Autodesk Fusion 360 part; units mm, degrees
(part 8 of 11)
  line L1134 (-0.172, -45.5718) -> (-0.1441, -45.6166)
  line L1135 (0.0223, -214.4938) -> (0.0013, -214.5276)
  line L1136 (14.483, -219.9371) -> (14.5191, -219.9534)
  line L1137 (-0.1969, -194.4741) -> (-0.2187, -194.5222)
  line L1138 (6.02, -212.839) -> (3.3593, -215.4997)
  line L1139 (0.0013, -194.5276) -> (-0.0174, -194.5626)
  line L1140 (14.4479, -219.9183) -> (14.483, -219.9371)
  line L1141 (-0.0683, -45.2866) -> (-0.0593, -45.3253)
  line L1142 (-0.0478, -45.3633) -> (-0.0338, -45.4005)
  line L1143 (19.8859, -185.7366) -> (19.9198, -185.7004)
  line L1144 (-0.2646, -214.6736) -> (-0.2732, -214.7258)
  line L1145 (14.7482, -220.1997) -> (18.42, -220.1997)
  line L1146 (9.713, -186.0997) -> (7.0807, -186.0997)
  line L1147 (-0.2786, -45.2189) -> (-0.2732, -45.2736)
  line L1148 (-0.0683, -214.7127) -> (-0.0748, -214.7519)
  line L1149 (19.9083, -185.2866) -> (19.9148, -185.2474)
  line L1150 (14.7514, -219.9997) -> (18.42, -219.9997)
  line L1151 (-0.0338, -214.5988) -> (-0.0478, -214.636)
  line L1152 (-0.0787, -45.2079) -> (-0.0748, -45.2474)
  line L1153 (14.4142, -219.8974) -> (14.4479, -219.9183)
  line L1154 (0.0454, -194.4616) -> (0.0223, -194.4938)
  line L1155 (-0.0748, -45.2474) -> (-0.0683, -45.2866)
  line L1156 (-0.1133, -45.6596) -> (-0.0798, -45.7004)
  line L1157 (14.3819, -219.8742) -> (14.4142, -219.8974)
  line L1158 (19.92, -218.4997) -> (19.92, -214.8311)
  line L1159 (-0.08, -45.0997) -> (-0.0787, -45.2079)
  line L1160 (0.0706, -45.5685) -> (0.0978, -45.5975)
  line L1161 (-0.28, -45.1009) -> (-0.2786, -45.2189)
  line L1162 (0.0454, -45.5378) -> (0.0706, -45.5685)
  line L1163 (-0.0593, -194.674) -> (-0.0683, -194.7127)
  line L1164 (-0.0798, -45.7004) -> (-0.0459, -45.7366)
  line L1165 (-0.2373, -194.5717) -> (-0.2526, -194.6222)
  line L1166 (-0.0798, -194.2989) -> (-0.1133, -194.3397)
  line L1167 (0.0978, -194.4019) -> (0.0706, -194.4308)
  line L1168 (14.3222, -219.8219) -> (14.3512, -219.849)
  line L1169 (0.0013, -45.4717) -> (0.0223, -45.5055)
  line L1170 (-0.0478, -194.636) -> (-0.0593, -194.674)
  line L1171 (-0.0683, -194.7127) -> (-0.0748, -194.7519)
  line L1172 (19.8574, -185.4367) -> (19.8738, -185.4005)
  line L1173 (9.713, -186.0997) -> (7.0807, -186.0997)
  line L1174 (14.594, -220.1843) -> (14.6461, -220.1929)
  line L1175 (14.7117, -219.9984) -> (14.7514, -219.9997)
  line L1176 (16.5635, -215.2997) -> (14.02, -212.7562)
  line L1177 (20.1186, -185.2189) -> (20.12, -185.1009)
  line L1178 (19.92, -218.4997) -> (19.92, -214.8311)
  line L1179 (19.8993, -185.3253) -> (19.9083, -185.2866)
  line L1180 (0.0223, -194.4938) -> (0.0013, -194.5276)
  line L1181 (-0.0478, -194.636) -> (-0.0593, -194.674)
  line L1182 (-0.2646, -194.6736) -> (-0.2732, -194.7258)
  line L1183 (-0.0338, -194.5988) -> (-0.0478, -194.636)
  line L1184 (9.7959, -185.8997) -> (7.1635, -185.8997)
  line L1185 (-0.0748, -194.7519) -> (-0.0787, -194.7914)
  line L1186 (20.12, -218.4997) -> (20.12, -214.8278)
  line L1187 (-0.1133, -194.3397) -> (-0.1441, -194.3827)
  line L1188 (6.02, -192.839) -> (3.3593, -195.4997)
  line L1189 (19.7946, -185.5378) -> (19.8177, -185.5055)
  line L1190 (3.6807, -182.6997) -> (1.72, -182.6997)
  circle A77 centre (9.92, -209.9997) radius 2.1
  arc A78 (13.1828, -217.9997) -> (12.9, -218.6825) centre (13.1828, -218.3997) ccw
  line L1191 (19.9198, -185.7004) -> (19.9533, -185.6596)
  line L1192 (1.72, -177.2997) -> (3.6807, -177.2997)
  line L1193 (19.8738, -185.4005) -> (19.8878, -185.3633)
  line L1194 (13.82, -210.1995) -> (13.6201, -209.9997)
  line L1195 (1.92, -182.4997) -> (1.92, -177.4997)
  line L1196 (1.72, -182.6997) -> (1.72, -177.2997)
  line L1197 (13.6201, -209.9997) -> (13.82, -209.7998)
  line L1198 (-0.1133, -214.3397) -> (-0.1441, -214.3827)
  line L1199 (-0.1441, -214.3827) -> (-0.172, -214.4275)
  line L1200 (-0.0683, -214.7127) -> (-0.0748, -214.7519)
  line L1201 (-0.0683, -194.7127) -> (-0.0748, -194.7519)
  line L1202 (20.0926, -185.3771) -> (20.1046, -185.3257)
  line L1203 (16.4807, -215.4997) -> (13.82, -212.839)
  line L1204 (-0.0459, -214.2627) -> (-0.0798, -214.2989)
  line L1205 (1.72, -182.6997) -> (1.72, -177.2997)
  line L1206 (19.9148, -185.2474) -> (19.9187, -185.2079)
  line L1207 (20.0587, -185.4771) -> (20.0773, -185.4277)
  line L1208 (14.02, -212.7562) -> (14.02, -210.1167)
  line L1209 (19.9148, -185.2474) -> (19.9187, -185.2079)
  line L1210 (-0.0787, -214.7914) -> (-0.08, -214.8997)
  line L1211 (19.8878, -185.3633) -> (19.8993, -185.3253)
  line L1212 (9.7981, -214.0997) -> (9.9208, -213.977)
  line L1213 (-0.2187, -194.5222) -> (-0.2373, -194.5717)
  line L1214 (-0.2786, -214.7804) -> (-0.28, -214.8985)
  line L1215 (0.0223, -194.4938) -> (0.0013, -194.5276)
  line L1216 (1.92, -177.4997) -> (3.7635, -177.4997)
  line L1217 (0.0978, -194.4019) -> (0.0706, -194.4308)
  line L1218 (3.7635, -182.4997) -> (1.92, -182.4997)
  line L1219 (-0.0787, -194.7914) -> (-0.08, -194.8997)
  line L1220 (-0.0787, -194.7914) -> (-0.08, -194.8997)
  line L1221 (-0.2373, -214.5717) -> (-0.2526, -214.6222)
  line L1222 (19.9533, -185.6596) -> (19.9841, -185.6166)
  line L1223 (10.127, -213.8997) -> (12.7593, -213.8997)
  line L1224 (0.0013, -194.5276) -> (-0.0174, -194.5626)
  line L1225 (-0.1969, -214.4741) -> (-0.2187, -214.5222)
  line L1226 (0.0706, -194.4308) -> (0.0454, -194.4616)
  line L1227 (14.02, -210.1167) -> (13.903, -209.9997)
  line L1228 (19.9083, -185.2866) -> (19.9148, -185.2474)
  line L1229 (-0.0338, -194.5988) -> (-0.0478, -194.636)
  line L1230 (20.1046, -185.3257) -> (20.1132, -185.2736)
  line L1231 (3.6807, -162.6997) -> (1.72, -162.6997)
  line L1232 (-0.0174, -194.5626) -> (-0.0338, -194.5988)
  line L1233 (-0.0478, -214.636) -> (-0.0593, -214.674)
  line L1234 (-0.172, -214.4275) -> (-0.1969, -214.4741)
  line L1235 (-0.0748, -194.7519) -> (-0.0787, -194.7914)
  line L1236 (0.0706, -214.4308) -> (0.0454, -214.4616)
  line L1237 (-0.0174, -214.5626) -> (-0.0338, -214.5988)
  line L1238 (9.7152, -213.8997) -> (9.92, -213.6949)
  line L1239 (-0.2732, -194.7258) -> (-0.2786, -194.7804)
  line L1240 (19.7694, -185.5685) -> (19.7946, -185.5378)
  circle A79 centre (9.92, -209.9997) radius 2.1
  line L1241 (0.0454, -194.4616) -> (0.0223, -194.4938)
  line L1242 (0.0706, -194.4308) -> (0.0454, -194.4616)
  line L1243 (19.8177, -185.5055) -> (19.8387, -185.4717)
  line L1244 (-0.0593, -214.674) -> (-0.0683, -214.7127)
  line L1245 (3.6807, -182.6997) -> (1.72, -182.6997)
  line L1246 (19.8387, -185.4717) -> (19.8574, -185.4367)
  line L1247 (13.903, -209.9997) -> (14.02, -209.8826)
  line L1248 (-0.0787, -214.7914) -> (-0.08, -214.8997)
  line L1249 (19.9187, -185.2079) -> (19.92, -185.0997)
  line L1250 (9.9208, -213.977) -> (10.0448, -214.0997)
  line L1251 (1.72, -177.2997) -> (3.6807, -177.2997)
  line L1252 (0.0978, -214.4019) -> (0.0706, -214.4308)
  line L1253 (10.127, -213.8997) -> (12.7593, -213.8997)
  line L1254 (1.2372, -192.9797) -> (-0.0459, -194.2627)
  arc A80 (13.1828, -218.1997) -> (13.0414, -218.5411) centre (13.1828, -218.3997) ccw
  line L1255 (1.72, -164.4997) -> (3.3593, -164.4997)
  line L1256 (-0.0593, -214.674) -> (-0.0683, -214.7127)
  line L1257 (3.7635, -202.4997) -> (1.92, -202.4997)
  line L1258 (1.92, -202.4997) -> (1.92, -197.4997)
  line L1259 (20.1132, -185.2736) -> (20.1186, -185.2189)
  line L1260 (14.1831, -219.9656) -> (14.2193, -219.9995)
  line L1261 (0.0013, -214.5276) -> (-0.0174, -214.5626)
  line L1262 (9.7152, -213.8997) -> (9.92, -213.6949)
  line L1263 (0.0454, -214.4616) -> (0.0223, -214.4938)
  line L1264 (-0.0798, -214.2989) -> (-0.1133, -214.3397)
  line L1265 (19.8738, -185.4005) -> (19.8878, -185.3633)
  line L1266 (-0.1441, -194.3827) -> (-0.172, -194.4275)
  line L1267 (20.0773, -185.4277) -> (20.0926, -185.3771)
  line L1268 (19.7694, -185.5685) -> (19.7946, -185.5378)
  line L1269 (1.72, -166.7368) -> (1.72, -164.4997)
  line L1270 (-0.0459, -194.2627) -> (-0.0798, -194.2989)
  line L1271 (-0.2526, -194.6222) -> (-0.2646, -194.6736)
  line L1272 (1.92, -166.7368) -> (1.92, -164.6997)
  arc A81 (1.3786, -166.8782) -> (1.72, -166.7368) centre (1.52, -166.7368) ccw
  line L1273 (13.82, -210.1995) -> (13.6201, -209.9997)
  line L1274 (-0.0478, -214.636) -> (-0.0593, -214.674)
  line L1275 (19.8993, -185.3253) -> (19.9083, -185.2866)
  line L1276 (20.012, -185.5718) -> (20.0369, -185.5252)
  line L1277 (19.8878, -185.3633) -> (19.8993, -185.3253)
  line L1278 (10.0448, -214.0997) -> (12.6765, -214.0997)
  line L1279 (19.8387, -185.4717) -> (19.8574, -185.4367)
  arc A82 (13.1828, -218.1997) -> (13.0414, -218.5411) centre (13.1828, -218.3997) ccw
  line L1280 (12.9, -218.6825) -> (14.1831, -219.9656)
  line L1281 (-0.0748, -214.7519) -> (-0.0787, -214.7914)
  line L1282 (13.6201, -209.9997) -> (13.82, -209.7998)
  line L1283 (19.9841, -185.6166) -> (20.012, -185.5718)
  line L1284 (3.6807, -202.6997) -> (1.72, -202.6997)
  line L1285 (0.0013, -214.5276) -> (-0.0174, -214.5626)
  line L1286 (3.2765, -164.6997) -> (5.82, -167.2432)
  line L1287 (19.9187, -185.2079) -> (19.92, -185.0997)
  line L1288 (3.6807, -162.6997) -> (1.72, -162.6997)
  line L1289 (1.92, -197.4997) -> (3.7635, -197.4997)
  line L1290 (19.8177, -185.5055) -> (19.8387, -185.4717)
  line L1291 (13.82, -212.839) -> (13.82, -210.1995)
  line L1292 (0.0978, -214.4019) -> (0.0706, -214.4308)
  line L1293 (-0.0748, -214.7519) -> (-0.0787, -214.7914)
  line L1294 (20.0369, -185.5252) -> (20.0587, -185.4771)
  arc A83 (1.3786, -166.8782) -> (1.72, -166.7368) centre (1.52, -166.7368) ccw
  line L1295 (19.8574, -185.4367) -> (19.8738, -185.4005)
  line L1296 (1.72, -197.2997) -> (3.6807, -197.2997)
  line L1297 (9.92, -213.6949) -> (10.127, -213.8997)
  line L1298 (-0.2732, -214.7258) -> (-0.2786, -214.7804)
  line L1299 (-0.2786, -194.7804) -> (-0.28, -194.8985)
  line L1300 (1.72, -202.6997) -> (1.72, -197.2997)
  line L1301 (9.92, -213.6949) -> (10.127, -213.8997)
  line L1302 (-0.2187, -214.5222) -> (-0.2373, -214.5717)
  line L1303 (-0.0338, -214.5988) -> (-0.0478, -214.636)
  line L1304 (13.82, -212.839) -> (13.82, -210.1995)
  line L1305 (0.0454, -214.4616) -> (0.0223, -214.4938)
  line L1306 (0.0706, -214.4308) -> (0.0454, -214.4616)
  line L1307 (19.7946, -185.5378) -> (19.8177, -185.5055)
  line L1308 (13.0414, -218.5411) -> (14.3222, -219.8219)
  line L1309 (-0.2526, -214.6222) -> (-0.2646, -214.6736)
  line L1310 (13.0414, -218.5411) -> (14.3222, -219.8219)
  line L1311 (1.72, -206.7368) -> (1.72, -204.4997)
  line L1312 (7.0807, -173.8997) -> (9.713, -173.8997)
  line L1313 (9.713, -166.0997) -> (7.0807, -166.0997)
  arc A84 (1.3786, -206.8782) -> (1.72, -206.7368) centre (1.52, -206.7368) ccw
  line L1314 (-0.2526, -185.3771) -> (-0.2373, -185.4277)
  line L1315 (18.12, -184.4997) -> (18.12, -186.7368)
  line L1316 (19.7422, -185.5975) -> (19.7694, -185.5685)
  line L1317 (16.4807, -215.4997) -> (13.82, -212.839)
  line L1318 (-0.0478, -185.3633) -> (-0.0338, -185.4005)
  arc A85 (17.92, -186.7368) -> (18.6028, -187.0197) centre (18.32, -186.7368) ccw
  line L1319 (15.42, -218.1997) -> (13.1828, -218.1997)
  line L1320 (1.72, -184.4997) -> (3.3593, -184.4997)
  line L1321 (1.3786, -213.1211) -> (0.0978, -214.4019)
  arc A86 (1.3786, -206.8782) -> (1.72, -206.7368) centre (1.52, -206.7368) ccw
  line L1322 (9.7959, -165.8997) -> (7.1635, -165.8997)
  line L1323 (-0.28, -185.1009) -> (-0.2786, -185.2189)
  line L1324 (1.2372, -212.9797) -> (-0.0459, -214.2627)
  line L1325 (-0.0174, -214.5626) -> (-0.0338, -214.5988)
  line L1326 (18.12, -184.4997) -> (18.12, -186.7368)
  line L1327 (6.02, -210.1995) -> (6.02, -212.839)
  line L1328 (17.92, -184.6997) -> (17.92, -186.7368)
  line L1329 (0.0223, -214.4938) -> (0.0013, -214.5276)
  line L1330 (-0.2187, -185.4771) -> (-0.1969, -185.5252)
  arc A87 (18.12, -186.7368) -> (18.4614, -186.8782) centre (18.32, -186.7368) ccw
  line L1331 (1.92, -184.6997) -> (3.2765, -184.6997)
  line L1332 (12.7593, -213.8997) -> (15.42, -216.5603)
  line L1333 (12.7593, -213.8997) -> (15.42, -216.5603)
  arc A88 (1.2372, -207.0197) -> (1.92, -206.7368) centre (1.52, -206.7368) ccw
  line L1334 (-0.172, -185.5718) -> (-0.1441, -185.6166)
  line L1335 (18.4614, -186.8782) -> (19.7422, -185.5975)
  line L1336 (3.2765, -204.6997) -> (5.82, -207.2432)
  line L1337 (1.72, -164.4997) -> (3.3593, -164.4997)
  line L1338 (1.3786, -213.1211) -> (0.0978, -214.4019)
  line L1339 (1.72, -166.7368) -> (1.72, -164.4997)
  line L1340 (12.6765, -214.0997) -> (15.22, -216.6432)
  line L1341 (1.92, -204.6997) -> (3.2765, -204.6997)
  line L1342 (1.72, -197.2997) -> (3.6807, -197.2997)
  line L1343 (18.4614, -186.8782) -> (19.7422, -185.5975)
  line L1344 (-0.2732, -185.2736) -> (-0.2646, -185.3257)
  line L1345 (5.82, -212.7562) -> (3.2765, -215.2997)
  line L1346 (-0.0338, -185.4005) -> (-0.0174, -185.4367)
  line L1347 (0.0978, -205.5975) -> (1.3786, -206.8782)
  line L1348 (1.72, -202.6997) -> (1.72, -197.2997)
  line L1349 (0.0223, -185.5055) -> (0.0454, -185.5378)
  line L1350 (4.42, -216.5603) -> (7.0807, -213.8997)
  line L1351 (3.3593, -164.4997) -> (6.02, -167.1603)
  line L1352 (-0.0748, -185.2474) -> (-0.0683, -185.2866)
  line L1353 (7.0807, -186.0997) -> (3.6807, -182.6997)
  line L1354 (15.22, -217.9997) -> (13.1828, -217.9997)
  line L1355 (3.3593, -164.4997) -> (6.02, -167.1603)
  line L1356 (6.02, -210.1995) -> (6.02, -212.839)
  line L1357 (7.0807, -166.0997) -> (3.6807, -162.6997)
  line L1358 (1.92, -164.6997) -> (3.2765, -164.6997)
  line L1359 (3.6807, -202.6997) -> (1.72, -202.6997)
  line L1360 (7.0807, -166.0997) -> (3.6807, -162.6997)
  line L1361 (15.42, -218.1997) -> (13.1828, -218.1997)
  line L1362 (7.1635, -165.8997) -> (3.7635, -162.4997)
  arc A89 (18.12, -186.7368) -> (18.4614, -186.8782) centre (18.32, -186.7368) ccw
  line L1363 (19.7422, -185.5975) -> (19.7694, -185.5685)
  line L1364 (18.6028, -187.0197) -> (19.8859, -185.7366)
  line L1365 (-0.2373, -185.4277) -> (-0.2187, -185.4771)
  line L1366 (3.7635, -197.4997) -> (7.1635, -194.0997)
  line L1367 (-0.2646, -185.3257) -> (-0.2526, -185.3771)
  line L1368 (1.72, -186.7368) -> (1.72, -184.4997)
  arc A90 (6.94, -218.6825) -> (6.6572, -217.9997) centre (6.6572, -218.3997) ccw
  line L1369 (7.0807, -186.0997) -> (3.6807, -182.6997)
  line L1370 (0.0013, -185.4717) -> (0.0223, -185.5055)
  line L1371 (5.5178, -219.8219) -> (6.7986, -218.5411)
  line L1372 (9.92, -186.3066) -> (9.713, -186.0997)
  line L1373 (-0.28, -214.8985) -> (-0.28, -218.4997)
  line L1374 (16.0765, -182.4997) -> (12.6765, -185.8997)
  arc A91 (6.7986, -218.5411) -> (6.6572, -218.1997) centre (6.6572, -218.3997) ccw
  line L1375 (1.72, -204.4997) -> (3.3593, -204.4997)
  line L1376 (4.62, -216.6432) -> (7.1635, -214.0997)
  line L1377 (0.0978, -205.5975) -> (1.3786, -206.8782)
  line L1378 (5.5178, -219.8219) -> (6.7986, -218.5411)
  line L1379 (3.6807, -197.2997) -> (7.0807, -193.8997)
  line L1380 (1.72, -206.7368) -> (1.72, -204.4997)
  line L1381 (-0.0683, -185.2866) -> (-0.0593, -185.3253)
  line L1382 (1.92, -206.7368) -> (1.92, -204.6997)
  line L1383 (13.82, -189.7998) -> (13.82, -187.1603)
  line L1384 (6.6572, -217.9997) -> (4.62, -217.9997)
  line L1385 (0.0978, -185.5975) -> (1.3786, -186.8782)
  line L1386 (7.1635, -185.8997) -> (3.7635, -182.4997)
  line L1387 (6.6572, -218.1997) -> (4.42, -218.1997)
  arc A92 (6.7986, -218.5411) -> (6.6572, -218.1997) centre (6.6572, -218.3997) ccw
  line L1388 (-0.0478, -165.3633) -> (-0.0338, -165.4005)
  line L1389 (4.62, -217.9997) -> (4.62, -216.6432)
  line L1390 (4.42, -218.1997) -> (4.42, -216.5603)
  line L1391 (-0.08, -214.8997) -> (-0.08, -218.4997)
  line L1392 (-0.0593, -165.3253) -> (-0.0478, -165.3633)
  line L1393 (-0.0787, -185.2079) -> (-0.0748, -185.2474)
  line L1394 (1.72, -204.4997) -> (3.3593, -204.4997)
  line L1395 (-0.2786, -185.2189) -> (-0.2732, -185.2736)
  line L1396 (-0.0174, -185.4367) -> (0.0013, -185.4717)
  line L1397 (-0.0478, -185.3633) -> (-0.0338, -185.4005)
  line L1398 (9.92, -186.0238) -> (9.7959, -185.8997)
  line L1399 (0.0013, -185.4717) -> (0.0223, -185.5055)
  line L1400 (7.0807, -206.0997) -> (3.6807, -202.6997)
  line L1401 (-0.0338, -165.4005) -> (-0.0174, -165.4367)
  line L1402 (10.0441, -185.8997) -> (9.92, -186.0238)
  line L1403 (-0.1133, -185.6596) -> (-0.0798, -185.7004)
  line L1404 (16.1593, -182.6997) -> (12.7593, -186.0997)
  line L1405 (-0.1441, -165.6166) -> (-0.1133, -165.6596)
  line L1406 (7.1635, -205.8997) -> (3.7635, -202.4997)
  line L1407 (12.6765, -185.8997) -> (10.0441, -185.8997)
  line L1408 (0.0223, -185.5055) -> (0.0454, -185.5378)
  line L1409 (1.72, -184.4997) -> (3.3593, -184.4997)
  line L1410 (-0.0683, -165.2866) -> (-0.0593, -165.3253)
  line L1411 (6.6572, -218.1997) -> (4.42, -218.1997)
  line L1412 (13.82, -190.1995) -> (13.6201, -189.9997)
  line L1413 (-0.1969, -185.5252) -> (-0.172, -185.5718)
  line L1414 (0.0706, -165.5685) -> (0.0978, -165.5975)
  line L1415 (1.92, -186.7368) -> (1.92, -184.6997)
  line L1416 (10.127, -186.0997) -> (9.92, -186.3066)
  line L1417 (-0.0683, -165.2866) -> (-0.0593, -165.3253)
  line L1418 (-0.08, -165.0997) -> (-0.0787, -165.2079)
  line L1419 (-0.1441, -185.6166) -> (-0.1133, -185.6596)
  line L1420 (0.0454, -185.5378) -> (0.0706, -185.5685)
  line L1421 (4.42, -218.1997) -> (4.42, -216.5603)
  line L1422 (13.82, -190.1995) -> (13.6201, -189.9997)
  line L1423 (-0.28, -165.1009) -> (-0.2786, -165.2189)
  line L1424 (-0.0787, -185.2079) -> (-0.0748, -185.2474)
  line L1425 (3.3593, -184.4997) -> (6.02, -187.1603)
  line L1426 (13.903, -189.9997) -> (14.02, -189.8826)
  line L1427 (-0.0787, -165.2079) -> (-0.0748, -165.2474)
  line L1428 (-0.0174, -185.4367) -> (0.0013, -185.4717)
  line L1429 (0.0978, -185.5975) -> (1.3786, -186.8782)
  line L1430 (5.6207, -219.9995) -> (5.6569, -219.9656)
  line L1431 (-0.0593, -185.3253) -> (-0.0478, -185.3633)
  line L1432 (5.2837, -219.9674) -> (5.3209, -219.9534)
  line L1433 (7.1635, -174.0997) -> (9.7959, -174.0997)
  line L1434 (-0.0478, -205.3633) -> (-0.0338, -205.4005)
  line L1435 (-0.2732, -205.2736) -> (-0.2646, -205.3257)
  line L1436 (14.02, -190.1167) -> (13.903, -189.9997)
  line L1437 (13.6201, -189.9997) -> (13.82, -189.7998)
  line L1438 (12.7593, -186.0997) -> (10.127, -186.0997)
  line L1439 (16.1593, -182.6997) -> (12.7593, -186.0997)
  line L1440 (-0.2373, -205.4277) -> (-0.2187, -205.4771)
  line L1441 (0.0454, -165.5378) -> (0.0706, -165.5685)
  line L1442 (-0.172, -165.5718) -> (-0.1441, -165.6166)
  line L1443 (-0.0174, -165.4367) -> (0.0013, -165.4717)
  line L1444 (4.42, -216.5603) -> (7.0807, -213.8997)
  line L1445 (13.82, -187.1603) -> (16.4807, -184.4997)
  line L1446 (3.2765, -184.6997) -> (5.82, -187.2432)
  line L1447 (0.0223, -165.5055) -> (0.0454, -165.5378)
  line L1448 (12.7593, -186.0997) -> (10.127, -186.0997)
  line L1449 (-0.2786, -205.2189) -> (-0.2732, -205.2736)
  line L1450 (-0.0593, -185.3253) -> (-0.0478, -185.3633)
  line L1451 (5.4455, -220.1165) -> (5.4921, -220.0916)
  line L1452 (-0.08, -214.8997) -> (-0.08, -218.4997)
  line L1453 (-0.0683, -205.2866) -> (-0.0593, -205.3253)
  line L1454 (-0.0787, -165.2079) -> (-0.0748, -165.2474)
  line L1455 (-0.1133, -165.6596) -> (-0.0798, -165.7004)
  line L1456 (-0.0748, -205.2474) -> (-0.0683, -205.2866)
  line L1457 (-0.0174, -205.4367) -> (0.0013, -205.4717)
  line L1458 (3.3593, -204.4997) -> (6.02, -207.1603)
  line L1459 (-0.0748, -165.2474) -> (-0.0683, -165.2866)
  line L1460 (-0.0459, -185.7366) -> (1.2372, -187.0197)
  line L1461 (-0.2187, -165.4771) -> (-0.1969, -165.5252)
  line L1462 (-0.08, -185.0997) -> (-0.0787, -185.2079)
  line L1463 (3.3593, -184.4997) -> (6.02, -187.1603)
  circle A93 centre (9.92, -189.9997) radius 2.1
  line L1464 (13.82, -189.7998) -> (13.82, -187.1603)
  line L1465 (-0.0338, -205.4005) -> (-0.0174, -205.4367)
  line L1466 (0.0706, -185.5685) -> (0.0978, -185.5975)
  line L1467 (5.0918, -220.1997) -> (5.1413, -220.198)
  line L1468 (-0.2526, -165.3771) -> (-0.2373, -165.4277)
  line L1469 (6.02, -192.839) -> (3.3593, -195.4997)
  line L1470 (-0.0748, -185.2474) -> (-0.0683, -185.2866)
  line L1471 (0.0223, -165.5055) -> (0.0454, -165.5378)
  line L1472 (-0.0798, -185.7004) -> (-0.0459, -185.7366)
  line L1473 (13.82, -187.1603) -> (16.4807, -184.4997)
  line L1474 (-0.08, -185.0997) -> (-0.0787, -185.2079)
  line L1475 (9.92, -186.3066) -> (9.713, -186.0997)
  line L1476 (-0.0683, -185.2866) -> (-0.0593, -185.3253)
  line L1477 (1.72, -186.7368) -> (1.72, -184.4997)
  line L1478 (-0.0748, -205.2474) -> (-0.0683, -205.2866)
  line L1479 (-0.0338, -185.4005) -> (-0.0174, -185.4367)
  line L1480 (-0.0174, -165.4367) -> (0.0013, -165.4717)
  line L1481 (0.0454, -185.5378) -> (0.0706, -185.5685)
  line L1482 (9.713, -166.0997) -> (7.0807, -166.0997)
  line L1483 (0.0706, -185.5685) -> (0.0978, -185.5975)
  circle A94 centre (9.92, -189.9997) radius 2.1
  line L1484 (14.02, -189.8826) -> (14.02, -187.2432)
  line L1485 (0.0454, -165.5378) -> (0.0706, -165.5685)
  line L1486 (14.02, -187.2432) -> (16.5635, -184.6997)
  line L1487 (-0.172, -205.5718) -> (-0.1441, -205.6166)
  line L1488 (-0.0593, -165.3253) -> (-0.0478, -165.3633)
  line L1489 (-0.2646, -205.3257) -> (-0.2526, -205.3771)
  line L1490 (13.6201, -189.9997) -> (13.82, -189.7998)
  line L1491 (10.127, -186.0997) -> (9.92, -186.3066)
  line L1492 (16.4807, -184.4997) -> (18.12, -184.4997)
  line L1493 (5.207, -219.988) -> (5.2457, -219.979)
  line L1494 (0.0706, -205.5685) -> (0.0978, -205.5975)
  line L1495 (-0.0748, -165.2474) -> (-0.0683, -165.2866)
  line L1496 (16.5635, -184.6997) -> (17.92, -184.6997)
  line L1497 (-0.0338, -165.4005) -> (-0.0174, -165.4367)
  line L1498 (-0.0593, -205.3253) -> (-0.0478, -205.3633)
  line L1499 (16.4807, -184.4997) -> (18.12, -184.4997)
  line L1500 (5.3921, -219.9183) -> (5.4258, -219.8974)
  line L1501 (3.6807, -197.2997) -> (7.0807, -193.8997)
  line L1502 (7.0807, -173.8997) -> (9.713, -173.8997)
  line L1503 (5.1678, -219.9945) -> (5.207, -219.988)
  line L1504 (12.7593, -146.0997) -> (10.127, -146.0997)
  line L1505 (10.0448, -145.8997) -> (9.9208, -146.0223)
  line L1506 (9.92, -146.3044) -> (9.7152, -146.0997)
  line L1507 (0.0223, -105.5055) -> (0.0454, -105.5378)
  line L1508 (-0.0593, -105.3253) -> (-0.0478, -105.3633)
  line L1509 (-0.172, -105.5718) -> (-0.1441, -105.6166)
  line L1510 (-0.0174, -105.4367) -> (0.0013, -105.4717)
  line L1511 (12.6765, -145.8997) -> (10.0448, -145.8997)
  line L1512 (-0.0787, -105.2079) -> (-0.0748, -105.2474)
  line L1513 (0.0454, -105.5378) -> (0.0706, -105.5685)
  line L1514 (9.9208, -146.0223) -> (9.7981, -145.8997)
  arc A95 (13.1828, -137.9997) -> (12.9, -138.6825) centre (13.1828, -138.3997) ccw
  arc A96 (13.0414, -141.4582) -> (13.1828, -141.7997) centre (13.1828, -141.5997) ccw
  line L1515 (0.0454, -105.5378) -> (0.0706, -105.5685)
  line L1516 (-0.2786, -105.2189) -> (-0.2732, -105.2736)
  line L1517 (0.0706, -105.5685) -> (0.0978, -105.5975)
  line L1518 (0.0013, -105.4717) -> (0.0223, -105.5055)
  line L1519 (10.127, -146.0997) -> (9.92, -146.3044)
  line L1520 (-0.0798, -105.7004) -> (-0.0459, -105.7366)
  line L1521 (-0.2187, -105.4771) -> (-0.1969, -105.5252)
  line L1522 (-0.2373, -105.4277) -> (-0.2187, -105.4771)
  line L1523 (14.1831, -140.0337) -> (12.9, -141.3168)
  line L1524 (14.02, -147.2432) -> (16.5635, -144.6997)
  line L1525 (-0.0593, -105.3253) -> (-0.0478, -105.3633)
  line L1526 (12.9, -138.6825) -> (14.1831, -139.9656)
  line L1527 (-0.28, -105.1009) -> (-0.2786, -105.2189)
  arc A97 (13.1828, -138.1997) -> (13.0414, -138.5411) centre (13.1828, -138.3997) ccw
  line L1528 (0.0013, -105.4717) -> (0.0223, -105.5055)
  line L1529 (15.42, -143.439) -> (12.7593, -146.0997)
  line L1530 (-0.0478, -105.3633) -> (-0.0338, -105.4005)
  line L1531 (-0.2646, -105.3257) -> (-0.2526, -105.3771)
  line L1532 (-0.2526, -105.3771) -> (-0.2373, -105.4277)
  line L1533 (9.92, -146.3044) -> (9.7152, -146.0997)
  arc A98 (12.9, -141.3168) -> (13.1828, -141.9997) centre (13.1828, -141.5997) ccw
  line L1534 (-0.0748, -105.2474) -> (-0.0683, -105.2866)
  line L1535 (-0.08, -105.0997) -> (-0.0787, -105.2079)
  line L1536 (10.127, -146.0997) -> (9.92, -146.3044)
  line L1537 (-0.08, -105.0997) -> (-0.0787, -105.2079)
  line L1538 (12.7593, -146.0997) -> (10.127, -146.0997)
  arc A99 (13.1828, -138.1997) -> (13.0414, -138.5411) centre (13.1828, -138.3997) ccw
  arc A100 (13.0414, -141.4582) -> (13.1828, -141.7997) centre (13.1828, -141.5997) ccw
  line L1539 (-0.0478, -105.3633) -> (-0.0338, -105.4005)
  line L1540 (-0.1441, -105.6166) -> (-0.1133, -105.6596)
  line L1541 (17.92, -202.4997) -> (16.0765, -202.4997)
  line L1542 (7.0807, -33.8997) -> (9.713, -33.8997)
  line L1543 (12.7593, -53.8997) -> (16.1593, -57.2997)
  line L1544 (7.1635, -54.0997) -> (9.7959, -54.0997)
  line L1545 (19.7422, -194.4019) -> (18.4614, -193.1211)
  line L1546 (19.7694, -34.4308) -> (19.7422, -34.4019)
  line L1547 (18.6028, -47.0197) -> (19.8859, -45.7366)
  line L1548 (-0.08, -14.8997) -> (-0.08, -25.0997)
  line L1549 (17.92, -197.4997) -> (17.92, -202.4997)
  line L1550 (18.12, -193.2625) -> (18.12, -195.4997)
  line L1551 (-0.28, -14.8985) -> (-0.28, -25.1009)
  line L1552 (18.12, -44.4997) -> (18.12, -46.7368)
  line L1553 (6.02, -207.1603) -> (6.02, -209.7998)
  line L1554 (19.7422, -45.5975) -> (19.7694, -45.5685)
  line L1555 (19.7422, -34.4019) -> (18.4614, -33.1211)
  line L1556 (18.4614, -46.8782) -> (19.7422, -45.5975)
  arc A101 (18.4614, -33.1211) -> (18.12, -33.2625) centre (18.32, -33.2625) ccw
  line L1557 (13.82, -209.7998) -> (13.82, -207.1603)
  line L1558 (19.8177, -34.4938) -> (19.7946, -34.4616)
  line L1559 (19.9841, -34.3827) -> (19.9533, -34.3397)
  line L1560 (20.12, -185.1009) -> (20.12, -174.8985)
  line L1561 (17.92, -44.6997) -> (17.92, -46.7368)
  arc A102 (18.12, -46.7368) -> (18.4614, -46.8782) centre (18.32, -46.7368) ccw
  line L1562 (18.12, -197.2997) -> (18.12, -202.6997)
  line L1563 (19.7422, -194.4019) -> (18.4614, -193.1211)
  line L1564 (19.7946, -34.4616) -> (19.7694, -34.4308)
  line L1565 (19.8177, -34.4938) -> (19.7946, -34.4616)
  line L1566 (19.7422, -45.5975) -> (19.7694, -45.5685)
  line L1567 (19.7694, -34.4308) -> (19.7422, -34.4019)
  line L1568 (19.7946, -34.4616) -> (19.7694, -34.4308)
  line L1569 (5.82, -207.2432) -> (5.82, -209.8826)
  line L1570 (18.12, -44.4997) -> (18.12, -46.7368)
  line L1571 (19.9198, -34.2989) -> (19.8859, -34.2627)
  line L1572 (18.12, -202.6997) -> (16.1593, -202.6997)
  line L1573 (16.0765, -197.4997) -> (17.92, -197.4997)
  line L1574 (16.1593, -197.2997) -> (18.12, -197.2997)
  line L1575 (12.6765, -54.0997) -> (16.0765, -57.4997)
  line L1576 (3.6807, -177.2997) -> (7.0807, -173.8997)
  arc A103 (18.12, -46.7368) -> (18.4614, -46.8782) centre (18.32, -46.7368) ccw
  line L1577 (16.1593, -202.6997) -> (12.7593, -206.0997)
  line L1578 (12.7593, -193.8997) -> (16.1593, -197.2997)
  line L1579 (12.7593, -173.8997) -> (16.1593, -177.2997)
  line L1580 (19.8859, -194.2627) -> (18.6028, -192.9797)
  line L1581 (20.012, -34.4275) -> (19.9841, -34.3827)
  line L1582 (18.12, -197.2997) -> (18.12, -202.6997)
  line L1583 (10.0441, -54.0997) -> (12.6765, -54.0997)
  line L1584 (16.4807, -55.4997) -> (13.82, -52.839)
  line L1585 (3.6807, -57.2997) -> (7.0807, -53.8997)
  arc A104 (18.4614, -33.1211) -> (18.12, -33.2625) centre (18.32, -33.2625) ccw
  line L1586 (19.8859, -34.2627) -> (18.6028, -32.9797)
  line L1587 (7.0807, -26.0997) -> (3.6807, -22.6997)
  line L1588 (19.7422, -34.4019) -> (18.4614, -33.1211)
  line L1589 (16.5635, -55.2997) -> (14.02, -52.7562)
  arc A105 (17.92, -46.7368) -> (18.6028, -47.0197) centre (18.32, -46.7368) ccw
  line L1590 (17.92, -195.2997) -> (16.5635, -195.2997)
  line L1591 (18.4614, -46.8782) -> (19.7422, -45.5975)
  line L1592 (18.12, -202.6997) -> (16.1593, -202.6997)
  line L1593 (16.1593, -197.2997) -> (18.12, -197.2997)
  line L1594 (13.6201, -29.9997) -> (13.82, -29.7998)
  line L1595 (1.72, -55.4997) -> (1.72, -53.2625)
  line L1596 (9.713, -33.8997) -> (9.92, -33.6927)
  line L1597 (12.7593, -53.8997) -> (16.1593, -57.2997)
  arc A106 (1.92, -53.2625) -> (1.2372, -52.9797) centre (1.52, -53.2625) ccw
  circle A107 centre (9.92, -29.9997) radius 2.1
  line L1598 (9.92, -53.9755) -> (10.0441, -54.0997)
  line L1599 (9.92, -33.6927) -> (10.127, -33.8997)
  arc A108 (1.72, -53.2625) -> (1.3786, -53.1211) centre (1.52, -53.2625) ccw
  line L1600 (10.127, -33.8997) -> (12.7593, -33.8997)
  circle A109 centre (9.92, -29.9997) radius 2.1
  line L1601 (9.92, -33.9755) -> (10.0441, -34.0997)
  line L1602 (19.7946, -205.5378) -> (19.8177, -205.5055)
  line L1603 (10.127, -33.8997) -> (12.7593, -33.8997)
  line L1604 (19.9533, -205.6596) -> (19.9841, -205.6166)
  line L1605 (3.3593, -55.4997) -> (1.72, -55.4997)
  line L1606 (13.903, -49.9997) -> (14.02, -49.8826)
  line L1607 (16.4807, -35.4997) -> (13.82, -32.839)
  line L1608 (19.8574, -205.4367) -> (19.8738, -205.4005)
  line L1609 (10.127, -53.8997) -> (12.7593, -53.8997)
  line L1610 (13.82, -32.839) -> (13.82, -30.1995)
  line L1611 (5.82, -52.7562) -> (3.2765, -55.2997)
  line L1612 (19.9148, -205.2474) -> (19.9187, -205.2079)
  line L1613 (14.02, -50.1167) -> (13.903, -49.9997)
  line L1614 (6.02, -50.1995) -> (6.02, -52.839)
  arc A110 (1.72, -53.2625) -> (1.3786, -53.1211) centre (1.52, -53.2625) ccw
  line L1615 (9.92, -33.6927) -> (10.127, -33.8997)
  line L1616 (19.7694, -214.4308) -> (19.7422, -214.4019)
  line L1617 (19.9148, -214.7519) -> (19.9083, -214.7127)
  line L1618 (18.12, -33.2625) -> (18.12, -35.4997)
  line L1619 (19.7946, -205.5378) -> (19.8177, -205.5055)
  line L1620 (13.82, -30.1995) -> (13.6201, -29.9997)
  line L1621 (3.6807, -57.2997) -> (7.0807, -53.8997)
  line L1622 (10.0441, -34.0997) -> (12.6765, -34.0997)
  line L1623 (20.1046, -214.6736) -> (20.0926, -214.6222)
  line L1624 (1.92, -55.2997) -> (1.92, -53.2625)
  line L1625 (9.7959, -34.0997) -> (9.92, -33.9755)
  line L1626 (6.02, -52.839) -> (3.3593, -55.4997)
  line L1627 (9.7959, -54.0997) -> (9.92, -53.9755)
  line L1628 (19.9187, -214.7914) -> (19.9148, -214.7519)
  line L1629 (6.02, -52.839) -> (3.3593, -55.4997)
  line L1630 (13.903, -29.9997) -> (14.02, -29.8826)
  line L1631 (3.7635, -57.4997) -> (7.1635, -54.0997)
  line L1632 (19.9148, -205.2474) -> (19.9187, -205.2079)
  line L1633 (3.2765, -55.2997) -> (1.92, -55.2997)
  line L1634 (13.6201, -29.9997) -> (13.82, -29.7998)
  line L1635 (14.02, -30.1167) -> (13.903, -29.9997)
  line L1636 (9.713, -53.8997) -> (9.92, -53.6927)
  line L1637 (9.713, -33.8997) -> (9.92, -33.6927)
  line L1638 (10.127, -53.8997) -> (12.7593, -53.8997)
  line L1639 (9.713, -53.8997) -> (9.92, -53.6927)
  line L1640 (13.82, -30.1995) -> (13.6201, -29.9997)
  line L1641 (3.3593, -55.4997) -> (1.72, -55.4997)
  line L1642 (1.92, -57.4997) -> (3.7635, -57.4997)
  line L1643 (9.92, -53.6927) -> (10.127, -53.8997)
  line L1644 (19.8387, -205.4717) -> (19.8574, -205.4367)
  line L1645 (14.02, -32.7562) -> (14.02, -30.1167)
  line L1646 (13.82, -32.839) -> (13.82, -30.1995)
  line L1647 (9.92, -53.6927) -> (10.127, -53.8997)
  line L1648 (20.0369, -214.4741) -> (20.012, -214.4275)
  line L1649 (19.8738, -214.5988) -> (19.8574, -214.5626)
  line L1650 (20.1132, -205.2736) -> (20.1186, -205.2189)
  line L1651 (1.72, -57.2997) -> (3.6807, -57.2997)
  line L1652 (19.9198, -205.7004) -> (19.9533, -205.6596)
  line L1653 (19.8387, -214.5276) -> (19.8177, -214.4938)
  line L1654 (6.02, -50.1995) -> (6.02, -52.839)
  line L1655 (16.4807, -55.4997) -> (13.82, -52.839)
  line L1656 (20.012, -205.5718) -> (20.0369, -205.5252)
  line L1657 (1.72, -55.4997) -> (1.72, -53.2625)
  line L1658 (19.7694, -205.5685) -> (19.7946, -205.5378)
  line L1659 (12.6765, -34.0997) -> (16.0765, -37.4997)
  line L1660 (19.7694, -205.5685) -> (19.7946, -205.5378)
  line L1661 (19.9198, -214.2989) -> (19.8859, -214.2627)
  line L1662 (14.02, -49.8826) -> (14.02, -47.2432)
  line L1663 (10.0441, -45.8997) -> (9.92, -46.0238)
  line L1664 (19.8738, -205.4005) -> (19.8878, -205.3633)
  line L1665 (-0.0593, -54.674) -> (-0.0683, -54.7127)
  line L1666 (19.8738, -205.4005) -> (19.8878, -205.3633)
  line L1667 (12.6765, -45.8997) -> (10.0441, -45.8997)
  line L1668 (-0.0748, -54.7519) -> (-0.0787, -54.7914)
  line L1669 (13.82, -50.1995) -> (13.6201, -49.9997)
  line L1670 (12.7593, -46.0997) -> (10.127, -46.0997)
  line L1671 (20.0587, -214.5222) -> (20.0369, -214.4741)
  line L1672 (19.8574, -214.5626) -> (19.8387, -214.5276)
  line L1673 (0.0706, -54.4308) -> (0.0454, -54.4616)
  line L1674 (20.0587, -34.5222) -> (20.0369, -34.4741)
  line L1675 (13.82, -49.7998) -> (13.82, -47.1603)
  line L1676 (20.0926, -205.3771) -> (20.1046, -205.3257)
  line L1677 (13.82, -47.1603) -> (16.4807, -44.4997)
  line L1678 (19.8878, -205.3633) -> (19.8993, -205.3253)
  line L1679 (19.8387, -205.4717) -> (19.8574, -205.4367)
  line L1680 (18.12, -33.2625) -> (18.12, -35.4997)
  line L1681 (19.9187, -205.2079) -> (19.92, -205.0997)
  line L1682 (20.1186, -205.2189) -> (20.12, -205.1009)
  line L1683 (16.4807, -35.4997) -> (13.82, -32.839)
  line L1684 (19.8738, -214.5988) -> (19.8574, -214.5626)
  line L1685 (19.8574, -205.4367) -> (19.8738, -205.4005)
  line L1686 (19.8859, -205.7366) -> (19.9198, -205.7004)
  line L1687 (19.8993, -205.3253) -> (19.9083, -205.2866)
  line L1688 (12.7593, -33.8997) -> (16.1593, -37.2997)
  line L1689 (19.8387, -34.5276) -> (19.8177, -34.4938)
  line L1690 (12.7593, -46.0997) -> (10.127, -46.0997)
  line L1691 (20.1046, -205.3257) -> (20.1132, -205.2736)
  line L1692 (19.9083, -205.2866) -> (19.9148, -205.2474)
  line L1693 (12.7593, -33.8997) -> (16.1593, -37.2997)
  line L1694 (13.82, -47.1603) -> (16.4807, -44.4997)
  line L1695 (20.0587, -205.4771) -> (20.0773, -205.4277)
  line L1696 (10.127, -46.0997) -> (9.92, -46.3066)
  line L1697 (19.9841, -214.3827) -> (19.9533, -214.3397)
  line L1698 (9.92, -46.3066) -> (9.713, -46.0997)
  line L1699 (19.8177, -205.5055) -> (19.8387, -205.4717)
  line L1700 (9.92, -46.3066) -> (9.713, -46.0997)
  line L1701 (19.9083, -214.7127) -> (19.8993, -214.674)
  line L1702 (10.127, -46.0997) -> (9.92, -46.3066)
  line L1703 (14.02, -47.2432) -> (16.5635, -44.6997)
  line L1704 (19.7946, -214.4616) -> (19.7694, -214.4308)
  line L1705 (19.9187, -205.2079) -> (19.92, -205.0997)
  line L1706 (20.1184, -214.7783) -> (20.1132, -214.7258)
  line L1707 (19.8387, -34.5276) -> (19.8177, -34.4938)
  line L1708 (19.8177, -205.5055) -> (19.8387, -205.4717)
  line L1709 (1.72, -57.2997) -> (3.6807, -57.2997)
  line L1710 (17.92, -33.2625) -> (17.92, -35.2997)
  line L1711 (13.6201, -49.9997) -> (13.82, -49.7998)
  line L1712 (19.8878, -214.636) -> (19.8738, -214.5988)
  line L1713 (16.5635, -35.2997) -> (14.02, -32.7562)
  line L1714 (-0.0787, -54.7914) -> (-0.08, -54.8997)
  line L1715 (19.92, -214.8311) -> (19.9187, -214.7914)
  line L1716 (19.9533, -214.3397) -> (19.9198, -214.2989)
  line L1717 (9.92, -46.0238) -> (9.7959, -45.8997)
  line L1718 (19.7422, -205.5975) -> (19.7694, -205.5685)
  line L1719 (20.0773, -205.4277) -> (20.0926, -205.3771)
  line L1720 (19.7694, -214.4308) -> (19.7422, -214.4019)
  line L1721 (20.0369, -205.5252) -> (20.0587, -205.4771)
  line L1722 (-0.0478, -54.636) -> (-0.0593, -54.674)
  line L1723 (13.6201, -49.9997) -> (13.82, -49.7998)
  line L1724 (-0.1133, -54.3397) -> (-0.1441, -54.3827)
  line L1725 (13.82, -49.7998) -> (13.82, -47.1603)
  line L1726 (19.7422, -205.5975) -> (19.7694, -205.5685)
  line L1727 (13.82, -50.1995) -> (13.6201, -49.9997)
  line L1728 (20.1132, -214.7258) -> (20.1046, -214.6736)
  line L1729 (13.82, -52.839) -> (13.82, -50.1995)
  circle A111 centre (9.92, -49.9997) radius 2.1
  line L1730 (-0.2187, -34.5222) -> (-0.2373, -34.5717)
  line L1731 (-0.2526, -54.6222) -> (-0.2646, -54.6736)
  line L1732 (19.8878, -205.3633) -> (19.8993, -205.3253)
  line L1733 (-0.0174, -54.5626) -> (-0.0338, -54.5988)
  line L1734 (14.02, -52.7562) -> (14.02, -50.1167)
  line L1735 (13.82, -52.839) -> (13.82, -50.1995)
  line L1736 (18.12, -55.4997) -> (16.4807, -55.4997)
  line L1737 (-0.0683, -54.7127) -> (-0.0748, -54.7519)
  line L1738 (-0.0683, -34.7127) -> (-0.0748, -34.7519)
  line L1739 (-0.2786, -54.7804) -> (-0.28, -54.8985)
  line L1740 (18.12, -55.4997) -> (16.4807, -55.4997)
  line L1741 (3.3593, -35.4997) -> (1.72, -35.4997)
  line L1742 (0.0013, -34.5276) -> (-0.0174, -34.5626)
  line L1743 (-0.0748, -54.7519) -> (-0.0787, -54.7914)
  line L1744 (19.8177, -214.4938) -> (19.7946, -214.4616)
  line L1745 (19.8574, -214.5626) -> (19.8387, -214.5276)
  arc A112 (17.92, -206.7368) -> (18.6028, -207.0197) centre (18.32, -206.7368) ccw
  line L1746 (19.92, -214.8311) -> (19.9187, -214.7914)
  line L1747 (19.9841, -205.6166) -> (20.012, -205.5718)
  line L1748 (0.0013, -34.5276) -> (-0.0174, -34.5626)
  line L1749 (16.1593, -57.2997) -> (18.12, -57.2997)
  line L1750 (1.72, -42.6997) -> (1.72, -37.2997)
  line L1751 (-0.2732, -54.7258) -> (-0.2786, -54.7804)
  line L1752 (0.0978, -54.4019) -> (0.0706, -54.4308)
  line L1753 (13.82, -207.1603) -> (16.4807, -204.4997)
  line L1754 (20.012, -214.4275) -> (19.9841, -214.3827)
  line L1755 (16.5635, -204.6997) -> (17.92, -204.6997)
  line L1756 (19.7946, -214.4616) -> (19.7694, -214.4308)
  line L1757 (19.9083, -214.7127) -> (19.8993, -214.674)
  line L1758 (19.8993, -205.3253) -> (19.9083, -205.2866)
  line L1759 (19.9148, -214.7519) -> (19.9083, -214.7127)
  line L1760 (16.5635, -44.6997) -> (17.92, -44.6997)
  line L1761 (16.1593, -57.2997) -> (18.12, -57.2997)
  line L1762 (3.2765, -35.2997) -> (1.92, -35.2997)
  line L1763 (16.4807, -44.4997) -> (18.12, -44.4997)
  line L1764 (-0.2526, -34.6222) -> (-0.2646, -34.6736)
  line L1765 (18.12, -204.4997) -> (18.12, -206.7368)
  line L1766 (19.8993, -214.674) -> (19.8878, -214.636)
  line L1767 (20.12, -214.8278) -> (20.1184, -214.7783)
  line L1768 (0.0223, -54.4938) -> (0.0013, -54.5276)
  line L1769 (19.8387, -214.5276) -> (19.8177, -214.4938)
  circle A113 centre (9.92, -49.9997) radius 2.1
  line L1770 (19.8993, -214.674) -> (19.8878, -214.636)
  line L1771 (19.9083, -205.2866) -> (19.9148, -205.2474)
  line L1772 (-0.0478, -34.636) -> (-0.0593, -34.674)
  line L1773 (20.0773, -214.5717) -> (20.0587, -214.5222)
  line L1774 (-0.0787, -54.7914) -> (-0.08, -54.8997)
  arc A114 (18.12, -206.7368) -> (18.4614, -206.8782) centre (18.32, -206.7368) ccw
  line L1775 (19.8878, -214.636) -> (19.8738, -214.5988)
  line L1776 (16.4807, -44.4997) -> (18.12, -44.4997)
  line L1777 (1.72, -37.2997) -> (3.6807, -37.2997)
  line L1778 (0.0978, -54.4019) -> (0.0706, -54.4308)
  line L1779 (-0.2646, -54.6736) -> (-0.2732, -54.7258)
  line L1780 (1.72, -42.6997) -> (1.72, -37.2997)
  line L1781 (19.8177, -214.4938) -> (19.7946, -214.4616)
  arc A115 (18.12, -206.7368) -> (18.4614, -206.8782) centre (18.32, -206.7368) ccw
  line L1782 (16.0765, -57.4997) -> (17.92, -57.4997)
  line L1783 (19.92, -205.0997) -> (19.92, -194.8997)
  line L1784 (1.92, -37.4997) -> (3.7635, -37.4997)
  line L1785 (3.7635, -42.4997) -> (1.92, -42.4997)
  line L1786 (-0.0478, -54.636) -> (-0.0593, -54.674)
  line L1787 (-0.2373, -34.5717) -> (-0.2526, -34.6222)
  line L1788 (-0.08, -174.8997) -> (-0.08, -185.0997)
  line L1789 (-0.0787, -34.7914) -> (-0.08, -34.8997)
  line L1790 (-0.0174, -54.5626) -> (-0.0338, -54.5988)
  line L1791 (-0.0338, -54.5988) -> (-0.0478, -54.636)
  line L1792 (7.0807, -213.8997) -> (9.7152, -213.8997)
  line L1793 (6.2199, -49.9997) -> (6.02, -50.1995)
  line L1794 (-0.0798, -54.2989) -> (-0.1133, -54.3397)
  line L1795 (-0.2646, -34.6736) -> (-0.2732, -34.7258)
  line L1796 (6.2199, -49.9997) -> (6.02, -50.1995)
  line L1797 (0.0454, -54.4616) -> (0.0223, -54.4938)
  line L1798 (3.6807, -42.6997) -> (1.72, -42.6997)
  line L1799 (1.92, -42.4997) -> (1.92, -37.4997)
  line L1800 (3.6807, -37.2997) -> (7.0807, -33.8997)
  line L1801 (5.82, -50.1167) -> (5.82, -52.7562)
  line L1802 (20.12, -205.1009) -> (20.12, -194.8985)
  line L1803 (12.7593, -173.8997) -> (16.1593, -177.2997)
  line L1804 (18.12, -213.2625) -> (18.12, -215.4997)
  line L1805 (17.92, -213.2625) -> (17.92, -215.2997)
  line L1806 (13.82, -207.1603) -> (16.4807, -204.4997)
  line L1807 (19.7422, -214.4019) -> (18.4614, -213.1211)
  line L1808 (-0.0748, -34.7519) -> (-0.0787, -34.7914)
  line L1809 (16.1593, -202.6997) -> (12.7593, -206.0997)
  line L1810 (0.0454, -54.4616) -> (0.0223, -54.4938)
  line L1811 (-0.1969, -54.4741) -> (-0.2187, -54.5222)
  line L1812 (17.92, -55.2997) -> (16.5635, -55.2997)
  line L1813 (16.4807, -204.4997) -> (18.12, -204.4997)
  arc A116 (18.6028, -212.9797) -> (17.92, -213.2625) centre (18.32, -213.2625) ccw
  line L1814 (17.92, -204.6997) -> (17.92, -206.7368)
  line L1815 (-0.0459, -54.2627) -> (-0.0798, -54.2989)
  line L1816 (3.6807, -177.2997) -> (7.0807, -173.8997)
  line L1817 (18.12, -213.2625) -> (18.12, -215.4997)
  line L1818 (-0.2187, -54.5222) -> (-0.2373, -54.5717)
  line L1819 (19.9187, -214.7914) -> (19.9148, -214.7519)
  line L1820 (18.4614, -206.8782) -> (19.7422, -205.5975)
  line L1821 (-0.0478, -34.636) -> (-0.0593, -34.674)
  line L1822 (18.12, -215.4997) -> (16.4807, -215.4997)
  line L1823 (1.72, -35.4997) -> (1.72, -33.2625)
  line L1824 (19.92, -205.0997) -> (19.92, -194.8997)
  line L1825 (-0.1441, -54.3827) -> (-0.172, -54.4275)
  line L1826 (14.02, -207.2432) -> (16.5635, -204.6997)
  line L1827 (18.6028, -207.0197) -> (19.8859, -205.7366)
  line L1828 (18.12, -215.4997) -> (16.4807, -215.4997)
  line L1829 (-0.0338, -54.5988) -> (-0.0478, -54.636)
  line L1830 (-0.172, -54.4275) -> (-0.1969, -54.4741)
  line L1831 (18.12, -204.4997) -> (18.12, -206.7368)
  line L1832 (16.4807, -204.4997) -> (18.12, -204.4997)
  line L1833 (-0.2786, -34.7804) -> (-0.28, -34.8985)
  line L1834 (18.4614, -206.8782) -> (19.7422, -205.5975)
  line L1835 (20.0926, -214.6222) -> (20.0773, -214.5717)
  line L1836 (-0.0593, -54.674) -> (-0.0683, -54.7127)
  line L1837 (-0.0174, -34.5626) -> (-0.0338, -34.5988)
  line L1838 (12.7593, -193.8997) -> (16.1593, -197.2997)
  line L1839 (3.6807, -42.6997) -> (1.72, -42.6997)
  line L1840 (3.3593, -35.4997) -> (1.72, -35.4997)
  line L1841 (0.0223, -34.4938) -> (0.0013, -34.5276)
  line L1842 (-0.2373, -54.5717) -> (-0.2526, -54.6222)
  line L1843 (-0.0338, -34.5988) -> (-0.0478, -34.636)
  line L1844 (0.0013, -54.5276) -> (-0.0174, -54.5626)
  line L1845 (-0.0593, -34.674) -> (-0.0683, -34.7127)
  line L1846 (5.82, -47.2432) -> (5.82, -49.8826)
  line L1847 (1.72, -37.2997) -> (3.6807, -37.2997)
  line L1848 (1.72, -35.4997) -> (1.72, -33.2625)
  line L1849 (0.0223, -54.4938) -> (0.0013, -54.5276)
  line L1850 (7.1635, -214.0997) -> (9.7981, -214.0997)
  line L1851 (1.3786, -53.1211) -> (0.0978, -54.4019)
  line L1852 (1.92, -44.6997) -> (3.2765, -44.6997)
  line L1853 (6.02, -32.839) -> (3.3593, -35.4997)
  line L1854 (12.6765, -194.0997) -> (16.0765, -197.4997)
  line L1855 (15.42, -216.5603) -> (15.42, -218.1997)
  line L1856 (12.6765, -174.0997) -> (16.0765, -177.4997)
  line L1857 (3.3593, -44.4997) -> (6.02, -47.1603)
  line L1858 (9.713, -193.8997) -> (9.92, -193.6927)
  line L1859 (19.92, -219.4997) -> (19.92, -218.4997)
  line L1860 (1.72, -44.4997) -> (3.3593, -44.4997)
  line L1861 (7.0807, -213.8997) -> (9.7152, -213.8997)
  line L1862 (1.3786, -53.1211) -> (0.0978, -54.4019)
  line L1863 (19.92, -185.0997) -> (19.92, -174.8997)
  line L1864 (1.2372, -52.9797) -> (-0.0459, -54.2627)
  line L1865 (9.713, -206.0997) -> (7.0807, -206.0997)
  line L1866 (-0.1441, -34.3827) -> (-0.172, -34.4275)
  line L1867 (18.42, -220.1997) -> (19.42, -220.1997)
  line L1868 (9.92, -206.3066) -> (9.713, -206.0997)
  line L1869 (7.0807, -193.8997) -> (9.713, -193.8997)
  arc A117 (19.42, -219.9997) -> (19.92, -219.4997) centre (19.42, -219.4997) ccw
  line L1870 (15.42, -216.5603) -> (15.42, -218.1997)
  line L1871 (-0.28, -174.8985) -> (-0.28, -185.1009)
  line L1872 (3.3593, -204.4997) -> (6.02, -207.1603)
  line L1873 (0.0013, -54.5276) -> (-0.0174, -54.5626)
  line L1874 (19.7422, -214.4019) -> (18.4614, -213.1211)
  arc A118 (18.4614, -213.1211) -> (18.12, -213.2625) centre (18.32, -213.2625) ccw
  line L1875 (0.0706, -54.4308) -> (0.0454, -54.4616)
  line L1876 (-0.0338, -34.5988) -> (-0.0478, -34.636)
  line L1877 (19.8859, -214.2627) -> (18.6028, -212.9797)
  line L1878 (5.82, -32.7562) -> (3.2765, -35.2997)
  line L1879 (17.92, -215.2997) -> (16.5635, -215.2997)
  line L1880 (-0.0593, -34.674) -> (-0.0683, -34.7127)
  line L1881 (1.72, -44.4997) -> (3.3593, -44.4997)
  line L1882 (10.127, -206.0997) -> (9.92, -206.3066)
  arc A119 (19.42, -219.9997) -> (19.92, -219.4997) centre (19.42, -219.4997) ccw
  line L1883 (0.0223, -34.4938) -> (0.0013, -34.5276)
  line L1884 (15.22, -216.6432) -> (15.22, -217.9997)
  line L1885 (6.02, -49.7998) -> (6.2199, -49.9997)
  line L1886 (-0.172, -34.4275) -> (-0.1969, -34.4741)
  line L1887 (-0.0787, -34.7914) -> (-0.08, -34.8997)
  line L1888 (-0.0683, -34.7127) -> (-0.0748, -34.7519)
  line L1889 (6.02, -47.1603) -> (6.02, -49.7998)
  line L1890 (19.92, -219.4997) -> (19.92, -218.4997)
  line L1891 (3.2765, -44.6997) -> (5.82, -47.2432)
  line L1892 (-0.0174, -34.5626) -> (-0.0338, -34.5988)
  line L1893 (-0.0748, -34.7519) -> (-0.0787, -34.7914)
  line L1894 (16.0765, -202.4997) -> (12.6765, -205.8997)
  line L1895 (-0.0798, -34.2989) -> (-0.1133, -34.3397)
  line L1896 (6.02, -49.7998) -> (6.2199, -49.9997)
  arc A120 (18.4614, -213.1211) -> (18.12, -213.2625) centre (18.32, -213.2625) ccw
  line L1897 (-0.2732, -34.7258) -> (-0.2786, -34.7804)
  line L1898 (-0.0683, -54.7127) -> (-0.0748, -54.7519)
  line L1899 (9.7959, -205.8997) -> (7.1635, -205.8997)
  line L1900 (9.92, -206.0238) -> (9.7959, -205.8997)
  line L1901 (-0.0459, -34.2627) -> (-0.0798, -34.2989)
  line L1902 (20.12, -219.4997) -> (20.12, -218.4997)
  line L1903 (7.0807, -193.8997) -> (9.713, -193.8997)
  line L1904 (0.0978, -34.4019) -> (0.0706, -34.4308)
  line L1905 (0.0706, -34.4308) -> (0.0454, -34.4616)
  line L1906 (6.02, -47.1603) -> (6.02, -49.7998)
  line L1907 (9.92, -206.3066) -> (9.713, -206.0997)
  line L1908 (0.0978, -45.5975) -> (1.3786, -46.8782)
  line L1909 (18.42, -219.9997) -> (19.42, -219.9997)
  line L1910 (14.483, -219.9371) -> (14.5191, -219.9534)
  line L1911 (9.7959, -194.0997) -> (9.92, -193.9755)
  line L1912 (14.2193, -219.9995) -> (14.2601, -220.033)
  line L1913 (6.02, -30.1995) -> (6.02, -32.839)
  arc A121 (1.2372, -47.0197) -> (1.92, -46.7368) centre (1.52, -46.7368) ccw
  line L1914 (3.3593, -44.4997) -> (6.02, -47.1603)
  line L1915 (6.2199, -29.9997) -> (6.02, -30.1995)
  line L1916 (6.02, -209.7998) -> (6.2199, -209.9997)
  line L1917 (18.42, -219.9997) -> (19.42, -219.9997)
  line L1918 (9.713, -193.8997) -> (9.92, -193.6927)
  line L1919 (10.0441, -205.8997) -> (9.92, -206.0238)
  arc A122 (1.3786, -46.8782) -> (1.72, -46.7368) centre (1.52, -46.7368) ccw
  line L1920 (0.0978, -45.5975) -> (1.3786, -46.8782)
  line L1921 (12.7593, -206.0997) -> (10.127, -206.0997)
  line L1922 (9.713, -206.0997) -> (7.0807, -206.0997)
  line L1923 (0.0454, -34.4616) -> (0.0223, -34.4938)
  line L1924 (5.82, -210.1167) -> (5.82, -212.7562)
  line L1925 (5.937, -209.9997) -> (5.82, -210.1167)
  line L1926 (12.6765, -205.8997) -> (10.0441, -205.8997)
  line L1927 (-0.1133, -34.3397) -> (-0.1441, -34.3827)
  line L1928 (1.3786, -33.1211) -> (0.0978, -34.4019)
  line L1929 (9.92, -193.6927) -> (10.127, -193.8997)
  arc A123 (1.72, -33.2625) -> (1.3786, -33.1211) centre (1.52, -33.2625) ccw
  arc A124 (19.42, -220.1997) -> (20.12, -219.4997) centre (19.42, -219.4997) ccw
  line L1930 (1.3786, -33.1211) -> (0.0978, -34.4019)
  line L1931 (1.72, -46.7368) -> (1.72, -44.4997)
  line L1932 (9.92, -193.6927) -> (10.127, -193.8997)
  arc A125 (1.72, -33.2625) -> (1.3786, -33.1211) centre (1.52, -33.2625) ccw
  line L1933 (0.0706, -34.4308) -> (0.0454, -34.4616)
  line L1934 (5.937, -49.9997) -> (5.82, -50.1167)
  line L1935 (-0.0459, -45.7366) -> (1.2372, -47.0197)
  line L1936 (0.0454, -34.4616) -> (0.0223, -34.4938)
  line L1937 (10.0441, -194.0997) -> (12.6765, -194.0997)
  line L1938 (10.127, -193.8997) -> (12.7593, -193.8997)
  line L1939 (10.127, -193.8997) -> (12.7593, -193.8997)
  arc A126 (1.3786, -46.8782) -> (1.72, -46.7368) centre (1.52, -46.7368) ccw
  line L1940 (7.1635, -194.0997) -> (9.7959, -194.0997)
  line L1941 (10.127, -206.0997) -> (9.92, -206.3066)
  line L1942 (1.72, -46.7368) -> (1.72, -44.4997)
  line L1943 (1.92, -46.7368) -> (1.92, -44.6997)
  line L1944 (1.2372, -32.9797) -> (-0.0459, -34.2627)
  line L1945 (6.02, -29.7998) -> (6.2199, -29.9997)
  line L1946 (14.3222, -219.8219) -> (14.3512, -219.849)
  line L1947 (0.0978, -34.4019) -> (0.0706, -34.4308)
  line L1948 (12.7593, -206.0997) -> (10.127, -206.0997)
  line L1949 (5.82, -49.8826) -> (5.937, -49.9997)
  line L1950 (5.82, -29.8826) -> (5.937, -29.9997)
  line L1951 (6.2199, -29.9997) -> (6.02, -30.1995)
  line L1952 (14.6722, -219.9945) -> (14.7117, -219.9984)
  line L1953 (5.937, -29.9997) -> (5.82, -30.1167)
  line L1954 (14.3512, -219.849) -> (14.3819, -219.8742)
  line L1955 (6.02, -209.7998) -> (6.2199, -209.9997)
  line L1956 (6.02, -29.7998) -> (6.2199, -29.9997)
  line L1957 (9.92, -193.9755) -> (10.0441, -194.0997)
  arc A127 (1.92, -33.2625) -> (1.2372, -32.9797) centre (1.52, -33.2625) ccw
  line L1958 (6.2199, -209.9997) -> (6.02, -210.1995)
  line L1959 (6.2199, -209.9997) -> (6.02, -210.1995)
  line L1960 (5.82, -209.8826) -> (5.937, -209.9997)
  line L1961 (5.82, -30.1167) -> (5.82, -32.7562)
  line L1962 (0.0454, -45.5378) -> (0.0706, -45.5685)
  line L1963 (14.4142, -219.8974) -> (14.4479, -219.9183)